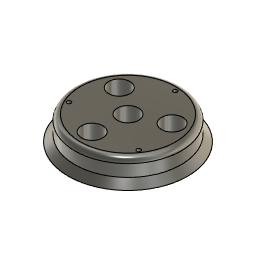
Anemometre-v1 (Autodesk Fusion 360 design; units mm, degrees)
Autodesk Fusion 360 part; units mm, degrees
sketch "Esquisse1" plane through (0, 0, 0) normal (0, 0, 1) x (1, 0, 0)
  circle A0 centre (0, 0) radius 40
  dimension "d1" = 80
  constraint coincident A0.centre origin
  measures "d1" diameter of A0
extrude "Extrusion1" add sketch "Esquisse1" along normal blind 18 makes body 1
sketch "Esquisse2" plane through (0, 0, 18) normal (0, 0, 1) x (-1, 0, 0)
  circle A0 centre (0, 0) radius 40
  circle A1 centre (0, 0) radius 8
  circle A2 centre (20.6567, -14.0819) radius 8
  circle A3 centre (-22.6458, -10.5909) radius 8
  circle A4 centre (2.0155, 25) radius 8
  circle A5 centre (-2.6573, -32.9619) radius 1.5
  circle A6 centre (30.0802, 14.3997) radius 1.5
  circle A7 centre (-27.459, 19.4091) radius 1.5
  dimension "d4" = 16
  dimension "d5" = 16
  dimension "d6" = 16
  dimension "d7" = 16
  dimension "d8" = 25
  dimension "d9" = 25
  dimension "d10" = 25
  dimension "d11" = 43.3
  dimension "d12" = 43.3
  dimension "d13" = 43.3026
  dimension "d14" = 3
  dimension "d15" = 3
  dimension "d16" = 3
  dimension "d17" = 30
  dimension "d18" = 30
  dimension "d19" = 30
  dimension "d20" = 30
  dimension "d21" = 30
  dimension "d22" = 30
  constraint coincident A0.centre A1.centre
  measures "d4" diameter of A1
  measures "d5" diameter of A2
  measures "d6" diameter of A3
  measures "d7" diameter of A4
  measures "d8" distance of A0.centre A2.centre
  measures "d9" distance of A0.centre A3.centre
  measures "d10" vertical distance of A0.centre A4.centre
  measures "d11" distance of A3.centre A4.centre
  measures "d12" distance of A2.centre A4.centre
  measures "d13" horizontal distance of A2.centre A3.centre
  measures "d14" diameter of A5
  measures "d15" diameter of A6
  measures "d16" diameter of A7
  measures "d17" distance of A2.centre A6.centre
  measures "d18" distance of A4.centre A6.centre
  measures "d19" distance of A4.centre A7.centre
  measures "d20" vertical distance of A3.centre A7.centre
  measures "d21" distance of A2.centre A5.centre
  measures "d22" distance of A3.centre A5.centre
extrude "Extrusion2" cut sketch "Esquisse2" against normal blind 18 contours A1 | A2 | A3 | A4 | A5 | A6 | A7 bodies 1
fillet "Congé1" radius 4 1 edges at (-37.2931, -14.4646, 18) on bodies 1
sketch "Esquisse3" plane through (0, 0, 0) normal (0, 0, -1) x (1, 0, 0)
  circle A0 centre (-2.0155, 25) radius 8
  circle A1 centre (-20.6567, -14.0819) radius 8
  circle A2 centre (2.6573, -32.9619) radius 1.5
  circle A3 centre (-30.0802, 14.3997) radius 1.5
  circle A4 centre (0, 0) radius 8
  circle A5 centre (22.6458, -10.5909) radius 8
  circle A6 centre (27.459, 19.4091) radius 1.5
  circle A7 centre (0, 0) radius 40
  circle A8 centre (0, 0) radius 45
  dimension "d27" = 90
  constraint concentric A4 A8
  measures "d27" diameter of A8
extrude "Extrusion3" add sketch "Esquisse3" against normal blind 5 separate body contours A8 makes body 2
chamfer "Chanfrein1" distance 5 angle 45 1 edges at (-41.9547, -16.2727, 5) on bodies 2
equation "d30 = 5 * mm"
